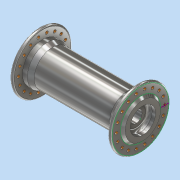
# Autodesk Inventor part: eje
Saved by Autodesk Inventor 2017 (Build 210142000, 142)
## iProperties
Part Number: eje
Material: Acero inoxidable
Document SubType Name: Modeling
Designer: Miguel A.
Density: 8 g/cm^3
Appearance: Cromo - Pulido
Author: Miguel A.
Autodesk Inventor part; units mm, degrees
ref_plane "YZ Plane" through (0, 0, 0) normal (1, 0, 0) x (0, 1, 0)
ref_plane "XZ Plane" through (0, 0, 0) normal (0, 1, 0) x (-1, 0, 0)
ref_plane "XY Plane" through (0, 0, 0) normal (0, 0, 1) x (1, 0, 0)
sketch "cubrebola" plane through (0, 0, 0) normal (0, 0, 1) x (1, 0, 0)
  line L0 (-57.0337, 12.8146) -> (-57.0337, 11.8146)
  arc A0 (-57.0337, 11.8146) -> (-53.5337, 8.3146) centre (-53.5337, 11.8146) ccw
  line L1 (-53.5337, 8.3146) -> (-49.0337, 8.3146)
  line L2 (-49.0337, 8.3146) -> (-49.0337, 2.3146)
  line L3 (-57.5337, 13.3146) -> (-65.0337, 13.3146)
  line L4 (-65.0337, 13.3146) -> (-65.0337, 2.3146)
  line L5 (-65.0337, 2.3146) -> (-49.0337, 2.3146)
  line L6 (-53.2763, 2.3146) -> (-52.9205, 2.3146)
  arc A1 (-57.0337, 12.8146) -> (-57.5337, 13.3146) centre (-57.5337, 12.8146) ccw
  line L7 (-65.0337, 6.3146) -> (-49.0337, 6.3146) construction
  point P0 (-57.0337, 13.3146)
  dimension "d26" = 8
  dimension "d27" = 11
  dimension "d28" = 6
  dimension "d29" = 3.5
  dimension "d36" = 8
  dimension "d38" = 0.5
  dimension "d43" = 4
  dimension "d44" = 16
  dimension "d45" = 2
  measures "d26" distance of point (-57.034, 13.315) L3.end
  measures "d27" distance of L3.end L4.end
  measures "d28" distance of L1.end L2.end
  measures "d29" radius of A0
  measures "d36" distance from line of L2 point (-57.034, 13.315)
  measures "d38" radius of A1
  measures "d43" distance between parallel lines of L5 L7
  measures "d44" distance of L7.start L7.end
  measures "d45" distance between parallel lines of L7 L1
sketch "bola eje" plane through (0, 0, 0) normal (0, 0, 1) x (1, 0, 0)
  circle A0 centre (-63.7612, 5.5387) radius 3.5
  dimension "d25" = 3.5
  measures "d25" radius of A0
sketch "eje" plane through (0, 0, 0) normal (0, 0, 1) x (1, 0, 0)
  line L0 (-50.226, 18.6479) -> (-45.226, 18.6479)
  line L1 (-45.226, 18.6479) -> (-40.226, 16.6479)
  line L2 (-48.726, 4.3979) -> (-1.726, 4.3979)
  line L3 (-1.726, 4.3979) -> (-1.726, 16.6479)
  line L4 (-55.726, 11.1479) -> (-55.726, 16.1479)
  line L5 (-55.726, 16.1479) -> (-53.226, 18.6479)
  line L6 (-53.226, 18.6479) -> (-53.226, 27.1479)
  arc A0 (-50.226, 27.1479) -> (-53.226, 27.1479) centre (-51.726, 27.1479) ccw
  line L7 (-50.226, 27.1479) -> (-50.226, 18.6479)
  line L8 (-40.226, 16.6479) -> (-1.726, 16.6479)
  line L9 (-55.726, 11.1479) -> (-52.226, 11.1479)
  arc A1 (-48.726, 7.6479) -> (-52.226, 11.1479) centre (-52.226, 7.6479) ccw
  line L10 (-48.726, 7.6479) -> (-48.726, 4.3979)
  line L11 (-85.079, -1.8521) -> (81.6269, -1.8521) construction
  point P0 (0, 0)
  point P1 (-47.726, 18.6479)
  point P2 (-1.726, 10.5229)
  point P3 (-1.726, -1.8521)
  dimension "d15" = 12.5
  dimension "d47" = 3
  dimension "d48" = 135
  dimension "d49" = 4
  dimension "d50" = 7
  dimension "d51" = 3.5
  dimension "d52" = 5
  dimension "d53" = 12
  dimension "d54" = 2
  dimension "d55" = 5
  dimension "d56" = 5
  dimension "d57" = 12.25
  dimension "d58" = 6.75
  dimension "d59" = 10
  dimension "d62" = 50
  measures "d15" diameter of L2 L11
  measures "d47" distance between parallel lines of L6 L7
  measures "d48" angle of L4 L5
  measures "d49" horizontal distance of L4.end A0.centre
  measures "d50" distance between parallel lines of L10 L4
  measures "d51" radius of A1
  measures "d52" distance of L4.start L4.end
  measures "d54" distance between parallel lines of L8 L0
  measures "d55" distance of L0.start L0.end
  measures "d56" horizontal distance of L1.end L0.end
  measures "d57" distance between parallel lines of L8 L2
  measures "d58" distance between parallel lines of L2 L9
  measures "d62" distance from line of A0.centre L3
derived "madre boceto.ipt"
sketch "Boceto1" plane through (0, 0, 0) normal (0, 0, 1) x (1, 0, 0)
  line L0 (-48.5, 20.5) -> (-43.5, 20.5)
  line L1 (-43.5, 20.5) -> (-38.5, 18.5)
  line L2 (-47, 6.25) -> (0, 6.25)
  line L3 (0, 6.25) -> (0, 18.5)
  line L4 (-54, 13) -> (-54, 18)
  line L5 (-54, 18) -> (-51.5, 20.5)
  line L6 (-51.5, 20.5) -> (-51.5, 29)
  arc A0 (-48.5, 29) -> (-51.5, 29) centre (-50, 29) ccw
  line L7 (-48.5, 29) -> (-48.5, 20.5)
  line L8 (-38.5, 18.5) -> (0, 18.5)
  line L9 (-54, 13) -> (-50.5, 13)
  arc A1 (-47, 9.5) -> (-50.5, 13) centre (-50.5, 9.5) ccw
  line L10 (-47, 9.5) -> (-47, 6.25)
  line L11 (-83.3529, 0) -> (83.3529, 0) construction
  point P0 (0, 0)
  constraints: 2 other
revolve "Revolución1" add sketch "Boceto1" angle 360 about axis through (-83.3529, 0, 0) along (1, 0, 0)
mirror "Simetría1" about plane through (0, 6.25, 0) normal (1, 0, 0) of "Revolución1"
sketch "Boceto2" plane through (51.5, 0, 0) normal (1, 0, 0) x (0, 0, -1)
  circle A0 centre (0, 0) radius 20.5 projected
  line L0 (0, 20.5) -> (0, 29)
  circle A1 centre (0, 0) radius 29 projected
  point P0 (0, 0)
  point P1 (0, 24.75)
  point P2 (0, 24.75)
  constraints: 2 end point, 2 vertical alignment, 1 coincident, 1 midpoint, 1 vertical, 2 other
hole "Agujero1" at (51.5, 24.75, 0) direction (-1, 0, 0) diameter 3 end through all
pattern_circular "Patrón circular1" count 18 over 360 about axis through (-23.5, 0, 0) along (1, 0, 0) of "Agujero1"
sketch "Boceto3" plane through (-51.5, 0, 0) normal (-1, 0, 0) x (0, 0, 1)
  circle A0 centre (0, 24.75) radius 1.5 projected
  circle A1 centre (0, 0) radius 20.5 projected
  line L0 (0, 23.25) -> (0, 26.25)
  circle A2 centre (0, 0) radius 29 projected
  point P0 (0, 0)
  constraints: 2 end point, 2 point on circle, 1 vertical
sketch "Boceto4" plane through (-48.5, 0, 0) normal (1, 0, 0) x (0, 0, -1)
  circle A0 centre (0, 24.75) radius 1.5 projected
  point P0 (0, 0)
sketch "Boceto5" plane through (48.5, 0, 0) normal (-1, 0, 0) x (0, 0, 1)
  circle A0 centre (0, 24.75) radius 1.5 projected
  point P0 (0, 0)
pattern_circular "Patrón circular2" count 18 over 360 about axis through (-19.25, 0, 0) along (-1, 0, 0)
